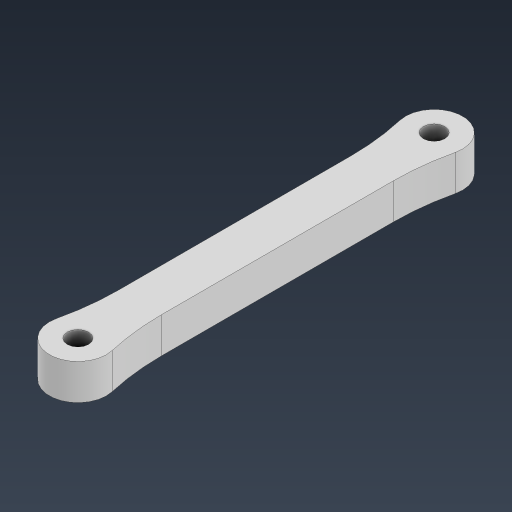
# Autodesk Inventor part: Connector
Saved by Autodesk Inventor 2024 (Build 280153000, 153)
## iProperties
Created: 2023-12-20
Part Number: Connector
Material: Generic
Document SubType Name: Modeling
Designer: Piter
Density: 1 g/cm^3
Appearance: Default
Author: Piter
Autodesk Inventor part; units mm, degrees
ref_plane "YZ Plane" through (0, 0, 0) normal (1, 0, 0) x (0, 1, 0)
ref_plane "XZ Plane" through (0, 0, 0) normal (0, 1, 0) x (-1, 0, 0)
ref_plane "XY Plane" through (0, 0, 0) normal (0, 0, 1) x (1, 0, 0)
sketch "Sketch1" plane through (0, 0, 0) normal (0, 1, 0) x (-1, 0, 0)
  circle A0 centre (0, 0) radius 4
  line L0 (0, 0) -> (0, -50)
  circle A1 centre (0, -50) radius 4
  line L1 (-3, -2.6458) -> (3, -2.6458)
  line L2 (3, -2.6458) -> (3, -47.3542)
  line L3 (3, -47.3542) -> (-3, -47.3542)
  line L4 (-3, -47.3542) -> (-3, -2.6458)
  line L5 (-3, -2.6458) -> (3, -47.3542) construction
  line L6 (3, -2.6458) -> (-3, -47.3542) construction
  circle A2 centre (0, 0) radius 1.5
  circle A3 centre (0, -50) radius 1.5
  point P0 (0, -25)
  dimension "d2" = 8
  dimension "d0" = 8
  dimension "d1" = 50
  dimension "d3" = 6
  dimension "d7" = 3
  dimension "d8" = 3
  constraints: 14 end point, 4 coincident, 3 centre point, 3 midpoint, 2 parallel, 1 horizontal, 1 perpendicular, 1 vertical, 3 other
  measures "d0" diameter of A0
  measures "d1" distance of L0.start L0.end
  measures "d3" distance of L2.end L3.end
  measures "d7" diameter of A2
  measures "d8" diameter of A3
extrude "Extrusion1" add sketch "Sketch1" along normal blind 5
fillet "Fillet1" radius 34.5 4 edges at (3, 2.5, -2.6458) (3, 2.5, -47.3542) (-3, 2.5, -2.6458) (-3, 2.5, -47.3542)
body "Solid1"
